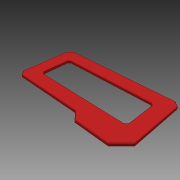
# Autodesk Inventor part: display_2004_frame
Saved by Autodesk Inventor 2014 (Build 180170000, 170)
## iProperties
Created: 2014-01-22
Part Number: display_2004_frame
Material: ABS Plastic
Document SubType Name: Modeling
Designer: buben
Density: 1.06 g/cm^3
Appearance: Light Red
Author: buben
Autodesk Inventor part; units mm, degrees
ref_plane "YZ Plane" through (0, 0, 0) normal (1, 0, 0) x (0, 1, 0)
ref_plane "XZ Plane" through (0, 0, 0) normal (0, 1, 0) x (-1, 0, 0)
ref_plane "XY Plane" through (0, 0, 0) normal (0, 0, 1) x (1, 0, 0)
sketch "Sketch1" plane through (0, 0, 0) normal (0, 1, 0) x (-1, 0, 0)
  line L0 (2, 0) -> (78, 0)
  line L1 (80, 2) -> (80, 25)
  line L2 (78, 27) -> (2, 27)
  line L3 (0, 25) -> (0, 2)
  line L4 (0, 25) -> (2, 27)
  line L5 (78, 27) -> (80, 25)
  line L6 (80, 2) -> (78, 0)
  line L7 (2, 0) -> (0, 2)
  line L8 (-8, 39) -> (88, 39)
  line L9 (92, 35) -> (92, -8)
  line L10 (88, -12) -> (-8, -12)
  line L11 (-12, -8) -> (-12, 35)
  line L12 (-12, 35) -> (-8, 39)
  line L13 (88, 39) -> (92, 35)
  line L14 (92, -8) -> (88, -12)
  line L15 (-8, -12) -> (-12, -8)
  point P0 (0, 0)
  point P1 (80, 27)
  point P2 (80, 0)
  point P3 (0, 27)
  point P4 (-12, 39)
  point P5 (92, -12)
  point P6 (92, 39)
  point P7 (-12, -12)
  point P8 (40, 39)
  point P9 (40, 27)
  point P10 (-12, 13.5)
  point P11 (0, 13.5)
  dimension "d0" = 2
  dimension "d1" = 2
  dimension "d2" = 2
  dimension "d3" = 2
  dimension "d4" = 2
  dimension "d5" = 2
  dimension "d6" = 2
  dimension "d7" = 2
  dimension "d8" = 80
  dimension "d9" = 27
  dimension "d10" = 4
  dimension "d11" = 4
  dimension "d12" = 4
  dimension "d13" = 4
  dimension "d14" = 4
  dimension "d15" = 4
  dimension "d16" = 4
  dimension "d17" = 4
  dimension "d18" = 12
  dimension "d19" = 12
  constraints: 32 end point, 16 point on line, 4 midpoint, 4 parallel, 2 horizontal, 2 perpendicular, 1 horizontal alignment, 1 vertical alignment
  measures "d0" distance of L3.start point (0, 27)
  measures "d1" distance of L2.end point (0, 27)
  measures "d2" distance of L2.start point (80, 27)
  measures "d3" distance of L1.end point (80, 27)
  measures "d4" distance of L1.start point (80, 0)
  measures "d5" distance of L0.end point (80, 0)
  measures "d6" distance of L0.start point (0, 0)
  measures "d7" distance of L3.end point (0, 0)
  measures "d8" distance between parallel lines of L1 L3
  measures "d9" distance between parallel lines of L0 L2
  measures "d10" distance of L11.end point (-12, 39)
  measures "d11" distance of L8.start point (-12, 39)
  measures "d12" distance of L8.end point (92, 39)
  measures "d13" distance of L9.start point (92, 39)
  measures "d14" distance of L9.end point (92, -12)
  measures "d15" distance of L10.start point (92, -12)
  measures "d16" distance of L10.end point (-12, -12)
  measures "d17" distance of L11.start point (-12, -12)
  measures "d18" distance between parallel lines of L3 L11
  measures "d19" distance between parallel lines of L2 L8
extrude "Extrusion1" add sketch "Sketch1" along normal blind 2
sketch "Sketch2" plane through (0, 2, 0) normal (0, 1, 0) x (1, 0, 0)
  line L0 (-92, -35) -> (-88, -39) projected
  line L1 (-88, -39) -> (8, -39) projected
  line L2 (8, -39) -> (2, -45)
  line L3 (2, -45) -> (-24, -45)
  line L4 (-24, -45) -> (-30, -39)
  point P0 (0, 0)
  dimension "d22" = 6
  dimension "d23" = 26
  constraints: 6 end point, 2 perpendicular, 1 parallel, 1 point on line
  measures "d22" distance between parallel lines of L1 L3
  measures "d23" distance of L2.end L3.end
extrude "Extrusion2" add sketch "Sketch2" against normal blind 2
chamfer "Chamfer1" distance 0.3 angle 45 18 edges at (-80, 2, 13.5) (-79, 2, 26) (-40, 2, 27) (-79, 2, 1) (-40, 2, 0) (-1, 2, 26) (0, 2, 13.5) (-1, 2, 1) (7, 2, 40) (12, 2, 13.5) (10, 2, -10) (-11, 2, 45) (-27, 2, 42) (-59, 2, 39) (-90, 2, 37) (-92, 2, 13.5) (-90, 2, -10) (-40, 2, -12)
equation "\"d1\" = d0"
equation "\"d2\" = d0"
equation "\"d3\" = d2"
equation "\"d4\" = d0"
equation "\"d5\" = d4"
equation "\"d6\" = d0"
equation "\"d7\" = d6"
equation "\"d11\" = d10"
equation "\"d12\" = d10"
equation "\"d13\" = d12"
equation "\"d14\" = d10"
equation "\"d15\" = d14"
equation "\"d16\" = d10"
equation "\"d17\" = d16"
equation "\"d19\" = d18"
body "Solid1"
